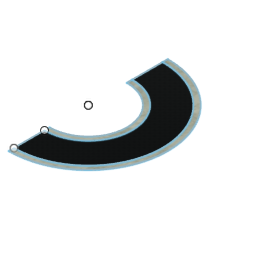
_New End Curve.09ecfdc2-4a22-4e7f-8e0c-03c076c3d32c (Autodesk Fusion 360 design; units mm, degrees)
Autodesk Fusion 360 part; units mm, degrees
sketch "sketch 351" plane through (0, 0, -2069.6955) normal (0, 0, 1) x (-1, 0, 0)
  arc A0 (2469.1082, 1963.9174) -> (2469.1082, -1002.6627) centre (2469.1082, 480.6274) ccw
  line L0 (2469.1082, -393.0627) -> (2469.1082, -1002.6627)
  arc A1 (2469.1082, 1354.3174) -> (2469.1082, -393.0627) centre (2469.1082, 480.6274) ccw
  line L1 (2469.1082, 1963.9174) -> (2469.1082, 1354.3174)
extrude "Extrude1" add sketch "sketch 351" along normal blind 6.35
sketch "sketch 377" plane through (0, 0, -2069.6955) normal (0, 0, 1) x (-1, 0, 0)
  arc A0 (2469.1082, 2065.5174) -> (2469.1082, -1104.2627) centre (2469.1082, 480.6274) ccw
  line L0 (2469.1082, -1002.6627) -> (2469.1082, -1104.2627)
  arc A1 (2469.1082, 1963.9174) -> (2469.1082, -1002.6627) centre (2469.1082, 480.6274) ccw
  line L1 (2469.1082, 2065.5174) -> (2469.1082, 1963.9174)
  arc A2 (2469.1082, 1354.3174) -> (2469.1082, -393.0627) centre (2469.1082, 480.6274) ccw
  line L2 (2469.1082, -291.4627) -> (2469.1082, -393.0627)
  arc A3 (2469.1082, 1252.7174) -> (2469.1082, -291.4627) centre (2469.1082, 480.6274) ccw
  line L3 (2469.1082, 1354.3174) -> (2469.1082, 1252.7174)
extrude "Extrude2" add sketch "sketch 377" along normal blind 6.096
